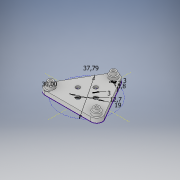
# Autodesk Inventor part: PlanetaryHolderTop
Saved by Autodesk Inventor 2018.3 (Build 223284000, 284)
## iProperties
Created: 2018-07-08
Part Number: PlanetaryHolderTop
Material: Generisch
Document SubType Name: Modeling
Designer: JochenAlt
Density: 1 g/cm^3
Appearance: Vorgabe
Author: JochenAlt
Autodesk Inventor part; units mm, degrees
ref_plane "YZ Plane" through (0, 0, 0) normal (1, 0, 0) x (0, 1, 0)
ref_plane "XZ Plane" through (0, 0, 0) normal (0, 1, 0) x (-1, 0, 0)
ref_plane "XY Plane" through (0, 0, 0) normal (0, 0, 1) x (1, 0, 0)
sketch "Skizze1" plane through (0, 0, 0) normal (0, 0, 1) x (1, 0, 0)
  circle A0 centre (0, 0) radius 18.895 construction
  circle A1 centre (0, 0) radius 9.5
  circle A2 centre (0, 18.895) radius 1
  line L0 (0, 0) -> (-16.3636, -9.4475) construction
  line L1 (0, 31.8099) -> (0, -27.3458) construction
  line L2 (-30.1836, 0) -> (30.1836, 0) construction
  circle A3 centre (0, 0) radius 6.35 construction
  circle A4 centre (0, 6.35) radius 1.5
  circle A5 centre (0, -6.35) radius 1.5
  circle A6 centre (6.35, 0) radius 1.5
  circle A7 centre (-6.35, 0) radius 1.5
  arc A8 (0, 22.895) -> (-3.4641, 20.895) centre (0, 18.895) ccw
  circle A9 centre (16.3636, -9.4475) radius 1
  arc A10 (16.3636, -13.4475) -> (19.8277, -7.4475) centre (16.3636, -9.4475) ccw
  circle A11 centre (-16.3636, -9.4475) radius 1
  arc A12 (-19.8277, -7.4475) -> (-16.3636, -13.4475) centre (-16.3636, -9.4475) ccw
  circle A13 centre (0, 18.895) radius 1.9
  circle A14 centre (16.3636, -9.4475) radius 1.9
  circle A15 centre (-16.3636, -9.4475) radius 1.9
  circle A16 centre (0, 18.895) radius 2.9
  circle A17 centre (16.3636, -9.4475) radius 2.9
  circle A18 centre (-16.3636, -9.4475) radius 2.9
  line L3 (-3.4641, 20.895) -> (-19.8277, -7.4475)
  line L4 (-16.3636, -13.4475) -> (16.3636, -13.4475)
  line L5 (3.4641, 20.895) -> (19.8277, -7.4475)
  arc A19 (3.4641, 20.895) -> (0, 22.895) centre (0, 18.895) ccw
  dimension "d0" = 37.79
  dimension "d1" = 2
  dimension "d2" = 30
  dimension "d3" = 19
  dimension "d4" = 12.7
  dimension "d5" = 3
  dimension "d8" = 3
  dimension "d26" = 3.8
  dimension "d27" = 1
  constraints: 20 centre point, 15 point on circle, 14 coincident, 12 equal radius, 8 end point, 7 tangent, 6 point on line, 1 symmetric about line
  measures "d0" diameter of A0
  measures "d1" diameter of A2
  measures "d2" angle of L0 L2
  measures "d3" diameter of A1
  measures "d4" diameter of A3
  measures "d5" diameter of A4
  measures "d8" radial gap between concentric circles of A2 A8
  measures "d26" diameter of A13
  measures "d27" radial gap between concentric circles of A16 A13
extrude "Extrusion1" add sketch "Skizze1" along normal blind 3 contours A1 | A19 L5 A10 L4 A12 L3 A8 | A13 | A14 | A15 | A16 | A17 | A18
extrude "Extrusion3" cut sketch "Skizze1" along normal blind 1.5 contours A1
extrude "Extrusion4" add sketch "Skizze1" along normal blind 2 from surface at 3 contours A13 | A14 | A15 | A16 | A17 | A18
extrude "Extrusion6" add sketch "Skizze1" along normal blind 2 from surface at 5 contours A13 | A14 | A15
extrude "Extrusion7" cut sketch "Skizze1" along normal blind 1.6 contours A13 | A14 | A15
